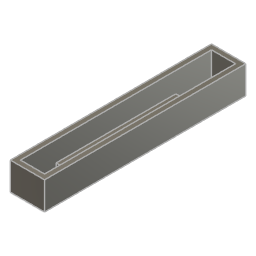
Slider Stand test v4 (Autodesk Fusion 360 design; units mm, degrees)
Autodesk Fusion 360 part; units mm, degrees
sketch "Sketch1" plane through (0, 0, 0) normal (0, 1, 0) x (1, 0, 0)
  line L0 (0, 0) -> (20.4, 0) construction
  line L1 (20.4, 0) -> (20.4, -88.85) construction
  line L2 (0, 0) -> (20.4, 0)
  line L3 (20.4, 0) -> (20.4, -88.85)
  line L4 (20.4, -88.85) -> (0, -88.85)
  line L5 (0, -88.85) -> (0, 0)
  line L6 (20.4, 0) -> (17.9, 0) construction
  line L7 (17.9, 0) -> (17.9, -2.5) construction
  line L8 (17.9, -2.5) -> (20.4, -2.5) construction
  line L9 (20.4, -2.5) -> (20.4, 0) construction
  circle A0 centre (17.9, -2.5) radius 1.5
  line L10 (0, 0) -> (2.5, 0) construction
  line L11 (2.5, 0) -> (2.5, -2.5) construction
  line L12 (2.5, -2.5) -> (0, -2.5) construction
  line L13 (0, -2.5) -> (0, 0) construction
  line L14 (0, -88.85) -> (2.5, -88.85) construction
  line L15 (2.5, -88.85) -> (2.5, -86.35) construction
  line L16 (2.5, -86.35) -> (0, -86.35) construction
  line L17 (0, -86.35) -> (0, -88.85) construction
  line L18 (20.4, -88.85) -> (17.9, -88.85) construction
  line L19 (17.9, -88.85) -> (17.9, -86.35) construction
  line L20 (17.9, -86.35) -> (20.4, -86.35) construction
  line L21 (20.4, -86.35) -> (20.4, -88.85) construction
  circle A1 centre (2.5, -86.35) radius 1.5
  circle A2 centre (17.9, -86.35) radius 1.5
  circle A3 centre (2.5, -2.5) radius 1.5
  circle A4 centre (2.5, -2.5) radius 2
  circle A5 centre (17.9, -2.5) radius 2
  circle A6 centre (2.5, -86.35) radius 2
  circle A7 centre (17.9, -86.35) radius 2
  dimension "d1" = 20.4
  dimension "d2" = 88.85
  dimension "d3" = 2.5
  dimension "d4" = 2.5
  dimension "d5" = 3
  dimension "d6" = 2.5
  dimension "d7" = 2.5
  dimension "d8" = 2.5
  dimension "d9" = 2.5
  dimension "d10" = 2.5
  dimension "d11" = 2.5
  dimension "d12" = 3
  dimension "d13" = 3
  dimension "d14" = 3
  dimension "d15" = 4
  dimension "d16" = 4
  dimension "d17" = 4
  dimension "d18" = 4
  constraint coincident L0.start L2.start
  constraint horizontal L0
  constraint perpendicular L0 L1
  constraint horizontal L2
  constraint vertical L3
  constraint horizontal L4
  constraint vertical L5
  constraint horizontal L6
  constraint vertical L7
  constraint horizontal L8
  constraint vertical L9
  constraint coincident L7.end L8.start
  constraint horizontal L10
  constraint vertical L11
  constraint horizontal L12
  constraint vertical L13
  constraint horizontal L14
  constraint vertical L15
  constraint horizontal L16
  constraint vertical L17
  constraint horizontal L18
  constraint vertical L19
  constraint horizontal L20
  constraint vertical L21
  constraint coincident L15.end L16.start
  constraint coincident L19 L20.start
  constraint coincident L11.end L12.start
  constraint concentric A3 A4
  constraint concentric A0 A5
  constraint concentric A1 A6
  constraint concentric A2 A7
  measures "d1" distance of L0.start L0.end
  measures "d2" distance of L0.end L1.end
  measures "d3" distance of L0.end L6.end
  measures "d4" distance of L0.end L8.end
  measures "d5" diameter of A0
  measures "d6" distance of L0.start L10.end
  measures "d7" distance of L0.start L12.end
  measures "d8" distance of L4.end L14.end
  measures "d9" distance of L4.end L16.end
  measures "d10" distance of L1.end L18.end
  measures "d11" distance of L1.end L20.end
  measures "d12" diameter of A1
  measures "d13" diameter of A2
  measures "d14" diameter of A3
  measures "d15" diameter of A4
  measures "d16" diameter of A5
  measures "d17" diameter of A6
  measures "d18" diameter of A7
extrude "Extrude1" add sketch "Sketch1" along normal blind 1 contours L2 L3 L4 L5 makes body 1
extrude "Extrude2" add sketch "Sketch1" along normal blind 1 contours A0 | A1 | A2 | A3 | A4 | A5 | A6 | A7 bodies 1
extrude "Extrude3" add sketch "Sketch1" along normal blind 10 contours A4 | A5 | A6 | A7 bodies 1
extrude "Extrude4" add 4 faces at (17.7887, 1, 3.5508) (2.9404, 1, 2.5827) (17.4222, 1, 86.4974) (2.3887, 1, 87.4008) along direction (0, 1, 0) blind 5 on bodies 1 bodies 1
sketch "Sketch2" plane through (0, 0, 0) normal (0, 1, 0) x (1, 0, 0)
  line L0 (55, 0) -> (64.5, 0) construction
  line L1 (55, 0) -> (55, -75.2) construction
  line L2 (55, -75.2) -> (64.5, -75.2)
  line L3 (64.5, -75.2) -> (64.5, 0)
  line L4 (64.5, 0) -> (55, 0)
  line L5 (55, 0) -> (55, -75.2)
  line L6 (64.5, -75.2) -> (68.5, -75.2) construction
  line L7 (68.5, -75.2) -> (68.5, -79.2) construction
  line L8 (68.5, -79.2) -> (64.5, -79.2) construction
  line L9 (64.5, -79.2) -> (64.5, -75.2) construction
  line L10 (55, 0) -> (51, 0) construction
  line L11 (51, 0) -> (51, 4) construction
  line L12 (51, 4) -> (55, 4) construction
  line L13 (55, 4) -> (55, 0) construction
  line L14 (51, 4) -> (68.5, 4)
  line L15 (68.5, 4) -> (68.5, -79.2)
  line L16 (68.5, -79.2) -> (51, -79.2)
  line L17 (51, -79.2) -> (51, 4)
  line L18 (59.75, -75.2) -> (59.75, -61.2) construction
  line L19 (59.75, 0) -> (59.75, -14) construction
  line L20 (59.75, -14) -> (55, -14) construction
  line L21 (59.75, -61.2) -> (64.5, -61.2) construction
  line L22 (55, -14) -> (64.5, -14)
  line L23 (64.5, -14) -> (64.5, -61.2)
  line L24 (64.5, -61.2) -> (55, -61.2)
  line L25 (55, -61.2) -> (55, -14)
  line L26 (55, -75.2) -> (64.5, -75.2)
  line L27 (64.5, -75.2) -> (64.5, -79.2)
  line L28 (64.5, -79.2) -> (55, -79.2)
  line L29 (55, -79.2) -> (55, -75.2)
  line L30 (55, 0) -> (64.5, 0)
  line L31 (64.5, 0) -> (64.5, 4)
  line L32 (64.5, 4) -> (55, 4)
  line L33 (55, 4) -> (55, 0)
  dimension "d27" = 9.5
  dimension "d28" = 75.2
  dimension "d29" = 4
  dimension "d30" = 4
  dimension "d31" = 4
  dimension "d32" = 4
  dimension "d35" = 14
  dimension "d36" = 14
  constraint horizontal L0
  constraint perpendicular L0 L1
  constraint horizontal L2
  constraint vertical L3
  constraint horizontal L4
  constraint vertical L5
  constraint horizontal L6
  constraint vertical L7
  constraint horizontal L8
  constraint vertical L9
  constraint horizontal L10
  constraint vertical L11
  constraint horizontal L12
  constraint vertical L13
  constraint horizontal L14
  constraint vertical L15
  constraint horizontal L16
  constraint vertical L17
  constraint midpoint L2 L18.start
  constraint perpendicular L2 L18
  constraint midpoint L4 L19.start
  constraint perpendicular L0 L19
  constraint coincident L1 L20.end
  constraint perpendicular L1 L20
  constraint coincident L3 L21.end
  constraint perpendicular L3 L21
  constraint horizontal L22
  constraint vertical L23
  constraint horizontal L24
  constraint vertical L25
  constraint horizontal L26
  constraint vertical L27
  constraint horizontal L28
  constraint vertical L29
  constraint horizontal L30
  constraint vertical L31
  constraint horizontal L32
  constraint vertical L33
  constraint coincident L14 L31.end
  measures "d27" distance of L0.start L0.end
  measures "d28" distance of L0.start L1.end
  measures "d29" distance of L2.end L6.end
  measures "d30" distance of L2.end L8.end
  measures "d31" distance of L0.start L10.end
  measures "d32" distance of L0.start L12.end
  measures "d35" distance of L18.start L18.end
  measures "d36" distance of L19.start L19.end
extrude "Extrude5" add sketch "Sketch2" along normal blind 1 separate body makes body 2
extrude "Extrude6" add sketch "Sketch2" along normal blind 10 contours L3 L5 L22 L23 L24 L25 bodies 2
extrude "Extrude7" add sketch "Sketch2" along normal blind 20 contours L5 L14 L16 L17 L25 L29 L33 | L3 L14 L15 L16 L23 L27 L31 bodies 2
sketch "Sketch3" plane through (0, 0, 0) normal (0, 1, 0) x (1, 0, 0)
  line L0 (85, -15) -> (94.5, -15)
  line L1 (94.5, -15) -> (94.5, -62.2)
  line L2 (94.5, -62.2) -> (85, -62.2)
  line L3 (85, -62.2) -> (85, -15)
  line L4 (94.5, -15) -> (96.5, -15)
  line L5 (96.5, -15) -> (96.5, -62.2)
  line L6 (96.5, -62.2) -> (94.5, -62.2)
  line L7 (94.5, -62.2) -> (94.5, -15)
  line L8 (85, -15) -> (83, -15)
  line L9 (83, -15) -> (83, -62.2)
  line L10 (83, -62.2) -> (85, -62.2)
  line L11 (85, -62.2) -> (85, -15)
  line L12 (85, -38.6) -> (85, -0.9) construction
  line L13 (94.5, -38.6) -> (94.5, -0.9) construction
  line L14 (85, -38.6) -> (85, -76.3) construction
  line L15 (94.5, -38.6) -> (94.5, -76.3) construction
  line L16 (83, -62.2) -> (85, -62.2)
  line L17 (85, -62.2) -> (85, -76.3)
  line L18 (85, -76.3) -> (83, -76.3)
  line L19 (83, -76.3) -> (83, -62.2)
  line L20 (94.5, -76.3) -> (96.5, -76.3)
  line L21 (96.5, -76.3) -> (96.5, -62.2)
  line L22 (96.5, -62.2) -> (94.5, -62.2)
  line L23 (94.5, -62.2) -> (94.5, -76.3)
  line L24 (83, -76.3) -> (96.5, -76.3)
  line L25 (96.5, -76.3) -> (96.5, -78.3)
  line L26 (96.5, -78.3) -> (83, -78.3)
  line L27 (83, -78.3) -> (83, -76.3)
  line L28 (85, -0.9) -> (83, -0.9)
  line L29 (83, -0.9) -> (83, -15)
  line L30 (83, -15) -> (85, -15)
  line L31 (85, -15) -> (85, -0.9)
  line L32 (94.5, -0.9) -> (96.5, -0.9)
  line L33 (96.5, -0.9) -> (96.5, -15)
  line L34 (96.5, -15) -> (94.5, -15)
  line L35 (94.5, -15) -> (94.5, -0.9)
  line L36 (96.5, -0.9) -> (83, -0.9)
  line L37 (83, -0.9) -> (83, 1.1)
  line L38 (83, 1.1) -> (96.5, 1.1)
  line L39 (96.5, 1.1) -> (96.5, -0.9)
  dimension "d41" = 9.5
  dimension "d42" = 47.2
  dimension "d43" = 2
  dimension "d44" = 2
  dimension "d49" = 37.7
  dimension "d50" = 37.7
  dimension "d51" = 37.7
  dimension "d52" = 37.7
  dimension "d53" = 2
  dimension "d54" = 2
  constraint horizontal L0
  constraint vertical L1
  constraint horizontal L2
  constraint vertical L3
  constraint horizontal L4
  constraint vertical L5
  constraint horizontal L6
  constraint vertical L7
  constraint horizontal L8
  constraint vertical L9
  constraint horizontal L10
  constraint vertical L11
  constraint midpoint L11 L12.start
  constraint parallel L11 L12
  constraint midpoint L7 L13.start
  constraint parallel L7 L13
  constraint parallel L3 L14
  constraint parallel L1 L15
  constraint horizontal L16
  constraint vertical L17
  constraint horizontal L18
  constraint vertical L19
  constraint horizontal L20
  constraint vertical L21
  constraint horizontal L22
  constraint vertical L23
  constraint horizontal L24
  constraint vertical L25
  constraint horizontal L26
  constraint vertical L27
  constraint horizontal L28
  constraint vertical L29
  constraint horizontal L30
  constraint vertical L31
  constraint horizontal L32
  constraint vertical L33
  constraint horizontal L34
  constraint vertical L35
  constraint horizontal L36
  constraint vertical L37
  constraint horizontal L38
  constraint vertical L39
  measures "d41" distance of L0.start L0.end
  measures "d42" distance of L0.start L2.end
  measures "d43" distance of L0.end L4.end
  measures "d44" distance of L0.start L8.end
  measures "d49" distance of L12.start L12.end
  measures "d50" distance of L13.start L13.end
  measures "d51" distance of L12.start L14.end
  measures "d52" distance of L13.start L15.end
  measures "d53" distance of L18.end L26.end
  measures "d54" distance of L32.end L38.end
extrude "Extrude8" add sketch "Sketch3" along normal blind 3 separate body contours L0 L1 L2 L3 L7 L11 makes body 3
extrude "Extrude9" add sketch "Sketch3" along normal blind 11 contours L3 L8 L9 L10 L11 L16 L30 | L1 L4 L5 L6 L7 L22 L34 bodies 3
extrude "Extrude10" add sketch "Sketch3" along normal blind 11 contours L8 L28 L29 L30 L31 L36 | L4 L32 L33 L34 L35 L36 | L10 L16 L17 L18 L19 L24 | L28 L32 L36 L37 L38 L39 | L6 L20 L21 L22 L23 L24 | L18 L20 L24 L25 L26 L27 bodies 3
hidden bodies 1 2
